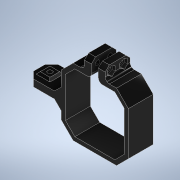
# Autodesk Inventor part: Montura motor para cadena
Saved by Autodesk Inventor 2022 (Build 260153000, 153)
## iProperties
Created: 2022-02-14
Part Number: Montura motor para cadena
Material: PET Plastic
Document SubType Name: Modeling
Designer: juanp
Density: 1.541 g/cm^3
Appearance: Polycarbonate - Clear
Author: juanp
Autodesk Inventor part; units mm, degrees
ref_plane "YZ Plane" through (0, 0, 0) normal (1, 0, 0) x (0, 1, 0)
ref_plane "XZ Plane" through (0, 0, 0) normal (0, 1, 0) x (-1, 0, 0)
sketch "Sketch1" plane through (0, 0, 0) normal (0, 0, 1) x (1, 0, 0)
  line L0 (21.15, -21.15) -> (14.4175, -21.15) construction
  line L1 (-21.15, -21.15) -> (-21.15, -14.4175) construction
  line L2 (-21.15, 21.15) -> (-14.4175, 21.15) construction
  line L3 (21.15, 21.15) -> (21.15, 14.4175) construction
  line L4 (21.15, -21.15) -> (-21.15, 21.15) construction
  line L5 (-21.15, -21.15) -> (21.15, 21.15) construction
  line L6 (-21.15, 14.4175) -> (-14.4175, 21.15) construction
  line L7 (14.4175, 21.15) -> (21.15, 14.4175) construction
  line L8 (21.15, -14.4175) -> (14.4175, -21.15) construction
  line L9 (-14.4175, -21.15) -> (-21.15, -14.4175) construction
  line L10 (-21.15, 14.4175) -> (-21.15, 21.15) construction
  line L11 (-14.4175, 21.15) -> (14.4175, 21.15) construction
  line L12 (14.4175, 21.15) -> (21.15, 21.15) construction
  line L13 (21.15, 14.4175) -> (21.15, -14.4175) construction
  line L14 (21.15, -14.4175) -> (21.15, -21.15) construction
  line L15 (14.4175, -21.15) -> (-14.4175, -21.15) construction
  line L16 (-14.4175, -21.15) -> (-21.15, -21.15) construction
  line L17 (-21.15, -14.4175) -> (-21.15, 14.4175) construction
  line L18 (-21.25, 14.4589) -> (-14.4589, 21.25)
  line L19 (-14.4589, 21.25) -> (14.4589, 21.25)
  line L20 (14.4589, 21.25) -> (21.25, 14.4589)
  line L21 (21.25, 14.4589) -> (21.25, -14.4589)
  line L22 (21.25, -14.4589) -> (14.4589, -21.25)
  line L23 (14.4589, -21.25) -> (-14.4589, -21.25)
  line L24 (-14.4589, -21.25) -> (-21.25, -14.4589)
  line L25 (-21.25, -14.4589) -> (-21.25, 14.4589)
  line L26 (-24.25, 15.7015) -> (-15.7015, 24.25)
  line L27 (-15.7015, 24.25) -> (15.7015, 24.25)
  line L28 (15.7015, 24.25) -> (24.25, 15.7015)
  line L29 (24.25, 15.7015) -> (24.25, -15.7015)
  line L30 (24.25, -15.7015) -> (15.7015, -24.25)
  line L31 (15.7015, -24.25) -> (-15.7015, -24.25)
  line L32 (-15.7015, -24.25) -> (-24.25, -15.7015)
  line L33 (-24.25, -15.7015) -> (-24.25, 15.7015)
  line L34 (-7.5, 21.25) -> (-2.5, 21.25)
  line L35 (-2.5, 21.25) -> (-2.5, 33.25)
  line L36 (-2.5, 33.25) -> (-7.5, 33.25)
  line L37 (-7.5, 33.25) -> (-7.5, 21.25)
  line L38 (2.5, 21.25) -> (7.5, 21.25)
  line L39 (7.5, 21.25) -> (7.5, 33.25)
  line L40 (7.5, 33.25) -> (2.5, 33.25)
  line L41 (2.5, 33.25) -> (2.5, 21.25)
  line L42 (-2.5, 27.25) -> (2.5, 27.25) construction
  line L43 (0, 27.25) -> (0, 21.15) construction
  point P0 (0, 0)
  point P1 (-17.7837, -17.7837)
  point P2 (-17.7837, 17.7837)
  point P3 (17.7837, 17.7837)
  point P4 (17.7837, -17.7837)
  point P5 (-7.5, 24.25)
  point P6 (7.5, 24.25)
  dimension "d0" = 42.3
  dimension "d1" = 42.3
  dimension "d2" = 50.3
  dimension "d3" = 0.1
  dimension "d4" = 3
  dimension "d5" = 5
  dimension "d6" = 5
  dimension "d7" = 9
  constraints: 88 end point, 26 parallel, 13 perpendicular, 10 midpoint, 9 point on line, 5 horizontal, 4 equal length, 1 collinear, 1 vertical, 14 other
  measures "d0" distance of L2.start L3.start
  measures "d1" distance of L1.start L2.start
  measures "d2" distance between parallel lines of L6 L8
  measures "d3" distance between parallel lines of L17 L25
  measures "d4" distance between parallel lines of L25 L33
  measures "d5" distance of L39.end L40.end
  measures "d6" distance between parallel lines of L41 L35
  measures "d7" distance between parallel lines of L40 L27
extrude "Extrusion1" add sketch "Sketch1" along normal blind 18 contours L25 L24 L23 L22 L21 L20 L19 L39 L27 L28 L29 L30 L31 L32 L33 L26 L37 L18 | L37 L27 L35 L19 | L37 L36 L35 L27 | L41 L27 L39 L19 | L41 L40 L39 L27
sketch "Sketch2" plane through (7.5, 24.25, 0) normal (1, 0, 0) x (0, 0, -1)
  line L0 (0, 0) -> (0, 9) projected
  line L1 (0, 9) -> (-18, 9) projected
  line L2 (-18, 0) -> (-18, 9) projected
  line L3 (0, 0) -> (-18, 0) projected
  line L4 (-18, 4.5) -> (-13.5, 4.5) construction
  line L5 (-4.5, 4.5) -> (0, 4.5) construction
  line L6 (0, 9) -> (0, -3) projected
  circle A0 centre (-13.5, 4.5) radius 1.65
  circle A1 centre (-4.5, 4.5) radius 1.65
  line L7 (-13.5, 4.5) -> (-9, 4.5) construction
  line L8 (-9, 4.5) -> (-4.5, 4.5) construction
  line L9 (-13.5, 1.2553) -> (-16.31, 2.8776)
  line L10 (-16.31, 2.8776) -> (-16.31, 6.1224)
  line L11 (-16.31, 6.1224) -> (-13.5, 7.7447)
  line L12 (-13.5, 7.7447) -> (-10.69, 6.1224)
  line L13 (-10.69, 6.1224) -> (-10.69, 2.8776)
  line L14 (-10.69, 2.8776) -> (-13.5, 1.2553)
  line L15 (-1.69, 2.8776) -> (-4.5, 1.2553)
  line L16 (-4.5, 1.2553) -> (-7.31, 2.8776)
  line L17 (-7.31, 2.8776) -> (-7.31, 6.1224)
  line L18 (-7.31, 6.1224) -> (-4.5, 7.7447)
  line L19 (-4.5, 7.7447) -> (-1.69, 6.1224)
  line L20 (-1.69, 6.1224) -> (-1.69, 2.8776)
  circle A2 centre (-13.5, 4.5) radius 4.5
  circle A3 centre (-4.5, 4.5) radius 4.5
  point P0 (0, -24.25)
  point P1 (-4.5, 0)
  point P2 (-13.5, 0)
  point P3 (-4.5, 9)
  point P4 (-13.5, 9)
  dimension "d10" = 3.3
  dimension "d11" = 5.62
  constraints: 32 end point, 5 coincident, 4 equal length, 3 point on line, 2 centre point, 2 horizontal, 2 vertical, 1 collinear, 1 equal radius, 1 midpoint, 1 perpendicular, 32 other
  measures "d10" diameter of A0
  measures "d11" distance between parallel lines of L10 L13
extrude "Extrusion2" cut sketch "Sketch2" against normal blind 15 contours A0 | A1
extrude "Extrusion4" cut sketch "Sketch2" against normal blind 2.35 contours L9 L10 L11 L12 L13 L14 | L15 L16 L17 L18 L19 L20
fillet "Fillet1" radius 3 4 edges at (-7.5, 24.25, 9) (2.5, 21.25, 9) (-2.5, 21.25, 9) (7.5, 24.25, 9)
chamfer "Chamfer1" distance 3 angle 45 4 edges at (-5, 33.25, 0) (5, 33.25, 0) (-5, 33.25, 18) (5, 33.25, 18)
ref_plane "Work Plane1" through (0, 0, 9) normal (0, 0, -1) x (-1, 0, 0)
sketch "Sketch4" plane through (0, 0, 0) normal (0, 0, -1) x (-1, 0, 0)
  line L0 (49.25, 0) -> (24.25, 0)
  line L1 (24.25, 0) -> (24.25, -5)
  line L2 (24.25, -5) -> (49.25, -5)
  line L3 (49.25, -5) -> (49.25, 0)
  line L4 (24.25, 15.7015) -> (24.25, -15.7015) projected
  point P0 (0, 0)
  dimension "d45" = 5
  dimension "d46" = 25
  constraints: 8 end point, 2 parallel, 1 horizontal, 1 midpoint, 1 perpendicular
  measures "d45" distance between parallel lines of L0 L2
  measures "d46" distance between parallel lines of L4 L3
extrude "Extrusion7" add sketch "Sketch4" against normal up to surface (18 mm away)
sketch "Sketch5" plane through (-49.25, 0, 0) normal (0, 1, 0) x (1, 0, 0)
  line L0 (0, -18) -> (25, -18) projected
  line L1 (25, 0) -> (25, -18) projected
  line L2 (0, 0) -> (25, 0) projected
  line L3 (0, 0) -> (0, -18) projected
  line L4 (25, 0) -> (25, -18) projected
  line L5 (25, -9) -> (7.8072, -9)
  line L6 (2.8072, -4) -> (12.8072, -4)
  line L7 (12.8072, -4) -> (12.8072, -14)
  line L8 (12.8072, -14) -> (2.8072, -14)
  line L9 (2.8072, -14) -> (2.8072, -4)
  line L10 (2.8072, -4) -> (12.8072, -14) construction
  line L11 (12.8072, -4) -> (2.8072, -14) construction
  circle A0 centre (7.8072, -9) radius 1.65
  point P0 (49.25, 0)
  dimension "d49" = 17.1928
  dimension "d50" = 10
  dimension "d51" = 10
  dimension "d54" = 3.3
  constraints: 14 end point, 3 midpoint, 2 horizontal, 2 parallel, 1 centre point, 1 coincident, 1 perpendicular
  measures "d49" distance of L5.start L5.end
  measures "d50" distance of L7.end L8.end
  measures "d51" distance of L6.end L7.end
  measures "d54" diameter of A0
extrude "Extrusion8" add sketch "Sketch5" along normal blind 1.5 contours L6 L7 L8 L9 | A0
extrude "Extrusion9" cut sketch "Sketch5" along normal through all both and the other way through all contours A0
chamfer "Chamfer5" distance 1.5 angle 45 4 edges at (-41.4428, 1.5, 14) (-46.4428, 1.5, 9) (-41.4428, 1.5, 4) (-36.4428, 1.5, 9)
chamfer "Chamfer6" distance 5 angle 45 4 edges at (-24.25, 0, 9) (-24.25, -5, 9) (-49.25, -2.5, 18) (-49.25, -2.5, 0)
sketch "Sketch6" plane through (-44.25, -5, 0) normal (0, -1, 0) x (1, 0, 0)
  circle A0 centre (2.8072, 9) radius 1.65 projected
  line L0 (-0.0028, 7.3776) -> (-0.0028, 10.6224)
  line L1 (-0.0028, 10.6224) -> (2.8072, 12.2447)
  line L2 (2.8072, 12.2447) -> (5.6172, 10.6224)
  line L3 (5.6172, 10.6224) -> (5.6172, 7.3776)
  line L4 (5.6172, 7.3776) -> (2.8072, 5.7553)
  line L5 (2.8072, 5.7553) -> (-0.0028, 7.3776)
  point P0 (44.25, 0)
  dimension "d63" = 5.62
  constraints: 12 end point, 1 coincident, 1 vertical, 13 other
  measures "d63" distance between parallel lines of L2 L5
extrude "Extrusion10" cut sketch "Sketch6" against normal blind 2.35 contours A0 | L0 L1 L2 L3 L4 L5
body "Solid1"
